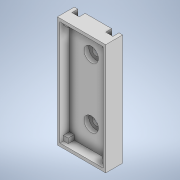
# Autodesk Inventor part: Arduinohalter
Saved by Autodesk Inventor 2021 (Build 250183000, 183)
## iProperties
Created: 2024-05-19
Part Number: Arduinohalter
Material: Generic
Document SubType Name: Modeling
Designer: Lukas
Density: 1 g/cm^3
Appearance: Default
Author: Lukas
Autodesk Inventor part; units mm, degrees
ref_plane "YZ Plane" through (0, 0, 0) normal (1, 0, 0) x (0, 1, 0)
ref_plane "XZ Plane" through (0, 0, 0) normal (0, 1, 0) x (-1, 0, 0)
ref_plane "XY Plane" through (0, 0, 0) normal (0, 0, 1) x (1, 0, 0)
sketch "Sketch1" plane through (0, 0, 0) normal (0, 0, 1) x (1, 0, 0)
  line L0 (-10, 23) -> (10, 23)
  line L1 (10, 23) -> (10, -23)
  line L2 (10, -23) -> (-10, -23)
  line L3 (-10, -23) -> (-10, 23)
  circle A0 centre (0, 12.5) radius 1.6
  circle A1 centre (0, -12.5) radius 1.6
  point P0 (0, 0)
  point P1 (0, 23)
  point P2 (-10, 0)
  dimension "d0" = 12.5
  dimension "d1" = 25
  dimension "d2" = 3.2
  dimension "d3" = 20
  dimension "d4" = 46
  constraints: 8 end point, 3 vertical alignment, 2 centre point, 2 midpoint, 2 parallel, 1 equal radius, 1 horizontal, 1 horizontal alignment, 1 perpendicular
  measures "d0" distance of point (0, 0) A1.centre
  measures "d1" distance of A0.centre A1.centre
  measures "d2" diameter of A0
  measures "d3" distance of L0.start L0.end
  measures "d4" distance of L0.end L1.end
extrude "Extrusion1" add sketch "Sketch1" along normal blind 3
sketch "Sketch2" plane through (0, 0, 3) normal (0, 0, 1) x (1, 0, 0)
  circle A0 centre (0, 12.5) radius 1.6 projected
  circle A1 centre (0, 12.5) radius 1.6 projected
  circle A2 centre (0, -12.5) radius 1.6 projected
  circle A3 centre (0, -12.5) radius 1.6 projected
  circle A4 centre (0, 12.5) radius 3
  circle A5 centre (0, -12.5) radius 3
  point P0 (0, 0)
  dimension "d7" = 6
  constraints: 2 centre point, 2 coincident, 1 equal radius
  measures "d7" diameter of A4
extrude "Extrusion2" cut sketch "Sketch2" against normal blind 2
sketch "Sketch3" plane through (0, 0, 3) normal (0, 0, 1) x (1, 0, 0)
  line L0 (-9, 21.75) -> (9, 21.75)
  line L1 (9, 21.75) -> (9, -21.75)
  line L2 (9, -21.75) -> (-9, -21.75)
  line L3 (-9, -21.75) -> (-9, 21.75)
  line L4 (-10, 23) -> (-10, -23) projected
  line L5 (10, 23) -> (-10, 23) projected
  line L6 (10, -23) -> (10, 23) projected
  line L7 (-10, -23) -> (10, -23) projected
  point P0 (0, 0)
  point P1 (-9, 0)
  point P2 (0, 21.75)
  dimension "d10" = 43.5
  dimension "d11" = 18
  constraints: 8 end point, 2 midpoint, 2 parallel, 1 horizontal, 1 horizontal alignment, 1 perpendicular, 1 vertical alignment
  measures "d10" distance of L0.end L1.end
  measures "d11" distance of L0.start L0.end
extrude "Extrusion3" add sketch "Sketch3" along normal blind 4
sketch "Sketch4" plane through (0, 0, 3) normal (0, 0, 1) x (1, 0, 0)
  line L0 (9, 21.75) -> (-9, 21.75) projected
  line L1 (-9, 21.75) -> (9, 21.75) projected
  line L2 (9, -21.75) -> (9, 21.75) projected
  line L3 (9, 21.75) -> (9, -21.75) projected
  line L4 (-9, 21.75) -> (-9, -21.75) projected
  line L5 (-9, -21.75) -> (-9, 21.75) projected
  line L6 (-9, -21.75) -> (9, -21.75) projected
  line L7 (9, -21.75) -> (-9, -21.75) projected
  line L8 (-9, 21.75) -> (-9, -21.75) projected
  line L9 (-9, 21.75) -> (-7, 21.75)
  line L10 (-7, 21.75) -> (-7, 19.75)
  line L11 (-7, 19.75) -> (-9, 19.75)
  line L12 (-9, 19.75) -> (-9, 21.75)
  line L13 (9, -21.75) -> (9, 21.75) projected
  line L14 (9, 21.75) -> (7, 21.75)
  line L15 (7, 21.75) -> (7, 19.75)
  line L16 (7, 19.75) -> (9, 19.75)
  line L17 (9, 19.75) -> (9, 21.75)
  line L18 (-9, -21.75) -> (9, -21.75) projected
  line L19 (9, -21.75) -> (7, -21.75)
  line L20 (7, -21.75) -> (7, -19.75)
  line L21 (7, -19.75) -> (9, -19.75)
  line L22 (9, -19.75) -> (9, -21.75)
  line L23 (-9, -21.75) -> (-7, -21.75)
  line L24 (-7, -21.75) -> (-7, -19.75)
  line L25 (-7, -19.75) -> (-9, -19.75)
  line L26 (-9, -19.75) -> (-9, -21.75)
  point P0 (0, 0)
  dimension "d14" = 2
  constraints: 32 end point, 8 parallel, 5 equal length, 4 horizontal, 4 perpendicular, 2 point on line
  measures "d14" distance of L10.end L11.end
extrude "Extrusion4" add sketch "Sketch4" along normal blind 2.5 contours L2 L16 L15 L0 | L10 L11 L4 L0 | L2 L6 L20 L21 | L25 L24 L6 L4
sketch "Sketch5" plane through (-10, 23, 0) normal (0, 1, 0) x (1, 0, 0)
  line L0 (20, 0) -> (0, 0) projected
  line L1 (0, 0) -> (0, -7) projected
  line L2 (20, -7) -> (0, -7) projected
  line L3 (20, 0) -> (20, -7) projected
  line L4 (0, 0) -> (0, -7) projected
  line L5 (20, 0) -> (0, 0) projected
  line L6 (18.5, 0) -> (15.5, 0)
  line L7 (15.5, 0) -> (15.5, -2.5)
  line L8 (15.5, -2.5) -> (18.5, -2.5)
  line L9 (18.5, -2.5) -> (18.5, 0)
  line L10 (4.5, 0) -> (1.5, 0)
  line L11 (1.5, 0) -> (1.5, -2.5)
  line L12 (1.5, -2.5) -> (4.5, -2.5)
  line L13 (4.5, -2.5) -> (4.5, 0)
  point P0 (10, 0)
  dimension "d25" = 1.5
  dimension "d26" = 3
  dimension "d27" = 2.5
  dimension "d28" = 1.5
  constraints: 16 end point, 4 parallel, 2 equal length, 2 horizontal, 2 perpendicular, 2 point on line
  measures "d25" distance between parallel lines of L3 L9
  measures "d26" distance of L7.end L8.end
  measures "d27" distance of L6.end L7.end
  measures "d28" distance between parallel lines of L1 L11
extrude "Extrusion5" cut sketch "Sketch5" against normal up to surface (46 mm away) contours L9 L8 L7 L0 | L13 L12 L11 L0
equation "\"d1\" = 2 * d0"
equation "\"d28\" = d25"
body "Solid1"
